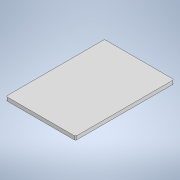
# Autodesk Inventor part: klapka1
Saved by Autodesk Inventor 2021 (Build 250183000, 183)
## iProperties
Created: 2025-11-23
Part Number: klapka1
Material: Ogólny
Document SubType Name: Modeling
Designer: humus
Density: 1 g/cm^3
Appearance: Domyślna
Author: humus
Autodesk Inventor part; units mm, degrees
ref_plane "YZ Plane" through (0, 0, 0) normal (1, 0, 0) x (0, 1, 0)
ref_plane "XZ Plane" through (0, 0, 0) normal (0, 1, 0) x (-1, 0, 0)
ref_plane "XY Plane" through (0, 0, 0) normal (0, 0, 1) x (1, 0, 0)
sketch "Szkic2" plane through (0, 0, 0) normal (0, 1, 0) x (-1, 0, 0)
  line L0 (0, 0) -> (-192, 0)
  line L1 (-192, 0) -> (-192, 272)
  line L2 (-192, 272) -> (0, 272)
  line L3 (0, 272) -> (0, 0)
  dimension "d0" = 192
  dimension "d1" = 272
  constraints: 8 end point, 2 parallel, 1 horizontal, 1 perpendicular
  measures "d0" distance of L1.end L2.end
  measures "d1" distance of L0.end L1.end
extrude "Wyciągnięcie proste1" add sketch "Szkic2" along normal mid plane 10
fillet "Zaokrąglenie1" radius 4 4 edges at (192, 0, 0) (0, 0, 0) (0, 0, 272) (192, 0, 272)
sketch "Szkic4" plane through (0, 0, 0) normal (0, 1, 0) x (-1, 0, 0)
  line L0 (-5, 5) -> (-187, 5)
  line L1 (-187, 5) -> (-187, 267)
  line L2 (-187, 267) -> (-5, 267)
  line L3 (-5, 267) -> (-5, 5)
  line L4 (-188, 0) -> (-4, 0) projected
  line L5 (0, 4) -> (0, 268) projected
  line L6 (-192, 268) -> (-192, 4) projected
  line L7 (-4, 272) -> (-188, 272) projected
  point P0 (0, 0)
  dimension "d13" = 5
  dimension "d14" = 5
  dimension "d16" = 5
  dimension "d17" = 5
  constraints: 8 end point, 2 parallel, 1 horizontal, 1 perpendicular
  measures "d13" distance between parallel lines of L4 L0
  measures "d14" distance between parallel lines of L5 L3
  measures "d16" distance between parallel lines of L6 L1
  measures "d17" distance between parallel lines of L7 L2
extrude "Wyciągnięcie proste3" cut sketch "Szkic4" against normal blind 5
